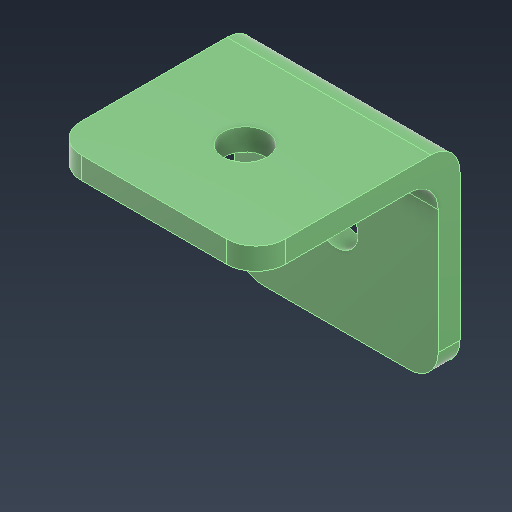
# Autodesk Inventor part: угол 25-26
Saved by Autodesk Inventor 2026 (Build 300175000, 175)
## iProperties
Created: 2025-11-01
Part Number: угол 25-26
Material: Типовые
Document SubType Name: Modeling
Designer: Phantom
Density: 1 g/cm^3
Appearance: Гладкий — темный травянисто-зеленый
Author: Phantom
Autodesk Inventor part; units mm, degrees
ref_plane "YZ Plane" through (0, 0, 0) normal (1, 0, 0) x (0, 1, 0)
ref_plane "XZ Plane" through (0, 0, 0) normal (0, 1, 0) x (-1, 0, 0)
ref_plane "XY Plane" through (0, 0, 0) normal (0, 0, 1) x (1, 0, 0)
sketch "Эскиз1" plane through (0, 0, 0) normal (0, 0, 1) x (1, 0, 0)
  line L0 (2, 0) -> (12, 0)
  line L1 (14, 2) -> (14, 14)
  line L2 (14, 14) -> (0, 14)
  line L3 (0, 14) -> (0, 2)
  circle A0 centre (7, 6.25) radius 1.5
  arc A1 (0, 2) -> (2, 0) centre (2, 2) ccw
  arc A2 (12, 0) -> (14, 2) centre (12, 2) ccw
  point P0 (0, 0)
  point P1 (14, 0)
  dimension "d0" = 14
  dimension "d1" = 14
  dimension "d2" = 3
  dimension "d5" = 2
  dimension "d14" = 7.75
  constraints: 8 end point, 4 point on circle, 4 point on line, 4 tangent, 3 centre point, 2 parallel, 1 equal radius, 1 horizontal, 1 perpendicular
  measures "d0" distance of L2.end L1.end
  measures "d1" distance of L1.end point (14, 0)
  measures "d2" diameter of A0
  measures "d5" radius of A1
  measures "d14" distance from line of L2 A0.centre
extrude "Выдавливание1" add sketch "Эскиз1" along normal blind 1.5
sketch "Эскиз2" plane through (0, 0, 1.5) normal (0, 0, 1) x (1, 0, 0)
  line L0 (14, 2) -> (14, 14) projected
  line L1 (14, 14) -> (0, 14)
  line L2 (0, 14) -> (0, 12.5)
  line L3 (0, 12.5) -> (14, 12.5)
  line L4 (14, 12.5) -> (14, 14)
  point P0 (0, 0)
  dimension "d6" = 14
  dimension "d7" = 1.5
  constraints: 8 end point, 2 parallel, 1 horizontal, 1 perpendicular
  measures "d6" distance of L3.end L2.end
  measures "d7" distance of L2.end L1.end
extrude "Выдавливание2" add sketch "Эскиз2" along normal blind 12.5
fillet "Сопряжение1" radius 2 4 edges at (0, 13.25, 14) (14, 13.25, 14) (7, 12.5, 1.5) (7, 14, 0)
sketch "Эскиз3" plane through (0, 12.5, 3.5) normal (0, -1, 0) x (1, 0, 0)
  line L0 (2, 10.5) -> (12, 10.5) projected
  line L1 (7, 10.5) -> (7, 9.5925)
  line L2 (0, 0) -> (0, 8.5) projected
  line L3 (0, 4.25) -> (2.1841, 4.25)
  circle A0 centre (7, 4.25) radius 1.5
  point P0 (0, -3.5)
  dimension "d11" = 3
  constraints: 4 end point, 2 midpoint, 1 centre point, 1 horizontal, 1 vertical
  measures "d11" diameter of A0
extrude "Выдавливание3" cut sketch "Эскиз3" against normal blind 12.5
